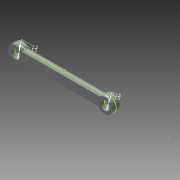
# Autodesk Inventor part: Shaft_Piston
Saved by Autodesk Inventor 2015 (Build 190159000, 159)
## iProperties
Created: 2016-07-06
Part Number: Shaft_Piston
Material: Generic
Document SubType Name: Modeling
Designer: Neelotpal Nag
Density: 1 g/cm^3
Appearance: Default
Mass: 0.0434138 g
Surface Area: 1.61026 cm^2
Volume: 0.0434138 cm^3
Author: Neelotpal Nag
Autodesk Inventor part; units mm, degrees
ref_plane "YZ Plane" through (0, 0, 0) normal (1, 0, 0) x (0, 1, 0)
ref_plane "XZ Plane" through (0, 0, 0) normal (0, 1, 0) x (-1, 0, 0)
ref_plane "XY Plane" through (0, 0, 0) normal (0, 0, 1) x (1, 0, 0)
sketch "Sketch4" plane through (0, 0, 0) normal (0, 0, 1) x (1, 0, 0)
  circle A0 centre (-12.5, 0) radius 0.75
  circle A1 centre (-12.5, 0) radius 1.25
  line L0 (-12.5, 0) -> (2.5, 0)
  circle A2 centre (2.5, 0) radius 0.75
  circle A3 centre (2.5, 0) radius 1.25
  line L1 (-12.5, 0.75) -> (2.5, 0.75)
  line L2 (-12.5, -0.75) -> (2.5, -0.75)
  point P0 (0, 0)
  point P1 (12.5, 0)
  dimension "d22" = 1.5
  dimension "d23" = 2.5
  dimension "d30" = 15
  dimension "d31" = 1.5
  dimension "d32" = 2.5
  constraints: 6 end point, 4 centre point, 4 coincident, 4 point on circle, 2 tangent, 1 horizontal
  measures "d22" diameter of A0
  measures "d23" diameter of A1
  measures "d30" distance of L0.start L0.end
  measures "d31" diameter of A2
  measures "d32" diameter of A3
extrude "Extrusion8" add sketch "Sketch4" along normal mid plane 1 contours L0 A1 L2 A0 | A0 L1 A1 L0 | L0 A3 L2 A1 | A1 L1 A3 L0 | A3 L1 A2 L0 | L0 A2 L2 A3
extrude "Extrusion9" add sketch "Sketch4" along normal mid plane 1.25 contours L0 A1 L2 A0 | A0 L1 A1 L0 | A0 L2 A1 L1 | A3 L1 A2 L0 | L0 A2 L2 A3 | A3 L2 A2 L1
body "Solid5"
